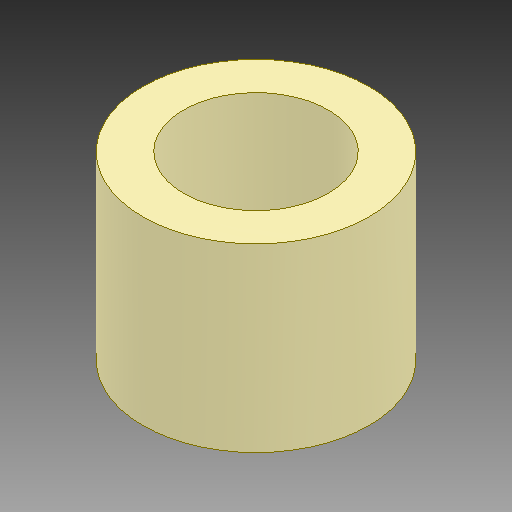
# Autodesk Inventor part: Nylon Abstandshalter 4mm D3.2
Saved by Autodesk Inventor 2019.1 (Build 231200000, 200)
## iProperties
Part Number: Nylon Abstandshalter 4mm D3.2
Material: Nylon 6/6
Document SubType Name: Modeling
Designer: rYan
Mass: 0.052398 g
Surface Area: 1.26229 cm^2
Volume: 0.0463699 cm^3
Density: 1.13 g/cm^3
Appearance: Nylon 6
Author: rYan
Autodesk Inventor part; units mm, degrees
ref_plane "YZ Plane" through (0, 0, 0) normal (1, 0, 0) x (0, 1, 0)
ref_plane "XZ Plane" through (0, 0, 0) normal (0, 1, 0) x (-1, 0, 0)
ref_plane "XY Plane" through (0, 0, 0) normal (0, 0, 1) x (1, 0, 0)
sketch "Skizze1" plane through (0, 0, 0) normal (0, 0, 1) x (1, 0, 0)
  circle A0 centre (0, 0) radius 1.6
  circle A1 centre (0, 0) radius 2.5
  dimension "d0" = 3.2
  dimension "d1" = 5
  constraints: 2 centre point, 2 coincident
  measures "d0" diameter of A0
  measures "d1" diameter of A1
extrude "Extrusion1" add sketch "Skizze1" along normal mid plane 4
